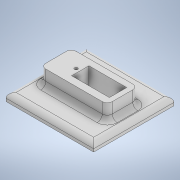
# Autodesk Inventor part: turret x
Saved by Autodesk Inventor 2020 (Build 240168000, 168)
## iProperties
Created: 2019-06-21
Part Number: turret x
Material: Generic
Document SubType Name: Modeling
Designer: kangh
Density: 1 g/cm^3
Appearance: Default
Author: kangh
Autodesk Inventor part; units mm, degrees
ref_plane "YZ Plane" through (0, 0, 0) normal (1, 0, 0) x (0, 1, 0)
ref_plane "XZ Plane" through (0, 0, 0) normal (0, 1, 0) x (-1, 0, 0)
ref_plane "XY Plane" through (0, 0, 0) normal (0, 0, 1) x (1, 0, 0)
sketch "Sketch1" plane through (0, 0, 0) normal (0, 1, 0) x (-1, 0, 0)
  line L0 (0, 0) -> (24, 0)
  line L1 (24, 0) -> (24, -11)
  line L2 (24, -11) -> (0, -11)
  line L3 (0, -11) -> (0, 0)
  line L4 (24, -11) -> (35.6612, -11)
  line L5 (35.6612, -11) -> (35.6612, 0)
  line L6 (35.6612, 0) -> (24, 0)
  line L7 (24, 0) -> (24, -11)
  line L8 (0, 0) -> (0, 20)
  line L9 (0, -11) -> (0, -31)
  line L10 (0, -31) -> (-10, -31)
  line L11 (-10, -31) -> (-10, 20)
  line L12 (-10, 20) -> (0, 20)
  line L13 (35.6612, 0) -> (45.6612, 0)
  line L14 (45.6612, 0) -> (45.6612, 20)
  line L15 (45.6612, 20) -> (0, 20)
  line L16 (45.6612, 0) -> (45.6612, -31)
  line L17 (45.6612, -31) -> (0, -31)
  line L18 (39.1081, 4.4818) -> (-3.116, 4.4818)
  line L19 (-3.116, 4.4818) -> (-3.116, -14.9069)
  line L20 (-3.116, -14.9069) -> (39.1081, -14.9069)
  line L21 (39.1081, -14.9069) -> (39.1081, 4.4818)
  dimension "d0" = 24
  dimension "d1" = 11
  dimension "d2" = 20
  dimension "d3" = 20
  dimension "d4" = 10
  dimension "d6" = 10
  constraints: 44 end point, 8 perpendicular, 6 parallel, 4 horizontal, 3 vertical, 1 point on line
  measures "d0" distance of L1.end L2.end
  measures "d1" distance of L0.end L1.end
  measures "d2" distance of L0.start L8.end
  measures "d3" distance of L2.end L9.end
  measures "d4" distance of L9.end L10.end
  measures "d6" distance of L5.end L13.end
extrude "Extrusion1" add sketch "Sketch1" along normal blind 15 contours L8 L18 L21 L13 L6 L0 | L3 L9 L20 L19 L18 L8 | L6 L5 L4 L1 | L2 L4 L5 L13 L21 L20 L9
extrude "Extrusion2" add sketch "Sketch1" along normal blind 5 contours L18 L19 L20 L9 L10 L11 L12 L8 | L8 L15 L14 L13 L21 L18 | L20 L21 L13 L16 L17 L9
fillet "Fillet1" radius 3.175 12 edges at (-17.8306, 5, 20) (10, 5, -5.5) (-17.8306, 5, -31) (-45.6612, 5, -5.5) (-17.996, 5, -14.9069) (-39.1081, 5, -5.2126) (-17.996, 5, 4.4818) (3.116, 5, -5.2126) (-39.1081, 10, -14.9069) (-39.1081, 10, 4.4818) (3.116, 10, -14.9069) (3.116, 10, 4.4818)
sketch "Sketch2" plane through (-45.6612, 0, -31) normal (-1, 0, 0) x (0, 0, 1)
  line L0 (51, 1.825) -> (0, 1.825) projected
  line L1 (20, 0) -> (31, 0) projected
  line L2 (23.2049, 1.825) -> (28.1129, 1.825)
  line L3 (28.1129, 1.825) -> (28.1129, 0)
  line L4 (28.1129, 0) -> (23.2049, 0)
  line L5 (23.2049, 0) -> (23.2049, 1.825)
  constraints: 8 end point, 2 parallel, 2 point on line, 1 horizontal, 1 perpendicular
extrude "Extrusion3" cut sketch "Sketch2" against normal blind 25
sketch "Sketch3" plane through (0, 15, 0) normal (0, 1, 0) x (1, 0, 0)
  line L0 (0, 0) -> (-24, 0) projected
  line L1 (-24, 11) -> (0, 11) projected
  line L2 (-24, 0) -> (-24, 11)
  line L3 (0, 11) -> (0, 0) projected
  line L4 (-24, 11) -> (0, 11)
  line L5 (0, 11) -> (0, 0)
  line L6 (0, 5.5) -> (2.5, 5.5)
  line L7 (-24, 2.8871) -> (-24, 7.7951) projected
  line L8 (-24, 5.3411) -> (-26.5, 5.3411)
  circle A0 centre (-26.5, 5.3411) radius 1
  dimension "d14" = 2.5
  dimension "d15" = 2.5
  dimension "d16" = 2
  constraints: 10 end point, 2 horizontal, 2 midpoint, 2 perpendicular, 1 centre point, 1 coincident, 1 collinear
  measures "d14" distance of L6.start L6.end
  measures "d15" distance of L8.start L8.end
  measures "d16" diameter of A0
extrude "Extrusion4" cut sketch "Sketch3" against normal blind 2.5 contours A0
body "Solid1"
